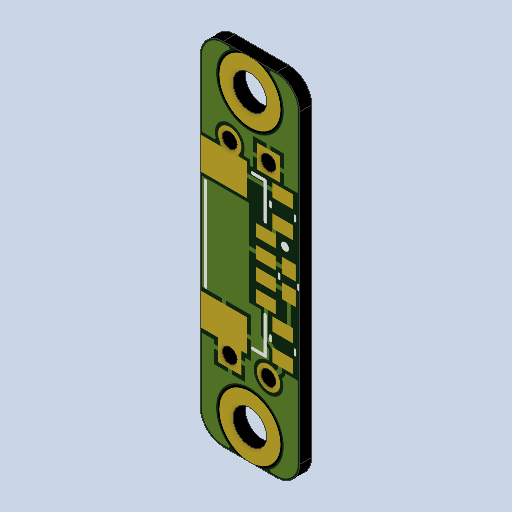
# Autodesk Inventor part: ND.ForageFeeder.BeamBreak_BOARD
Saved by Autodesk Inventor 2023.2 (Build 272271000, 271)
## iProperties
Created: 2021-12-10
Part Number: ND.ForageFeeder.BeamBreak_BOARD
Material: Generic
Document SubType Name: Modeling
Designer: Graeme
Density: 1 g/cm^3
Appearance: BoardColor
Author: Graeme
Autodesk Inventor part; units mm, degrees
ref_plane "YZ Plane" through (0, 0, 0) normal (1, 0, 0) x (0, 1, 0)
ref_plane "XZ Plane" through (0, 0, 0) normal (0, 1, 0) x (-1, 0, 0)
ref_plane "BoardFrontPlane" through (0, 0, 0) normal (0, 0, 1) x (1, 0, 0)
sketch "Sketch1" plane through (0, 0, 0) normal (0, 0, 1) x (1, 0, 0)
  line L0 (24, 22.5) -> (24, 42.5)
  arc A0 (25.5, 44) -> (24, 42.5) centre (25.5, 42.5) ccw
  line L1 (25.5, 44) -> (29, 44)
  arc A1 (30.5, 42.5) -> (29, 44) centre (29, 42.5) ccw
  line L2 (30.5, 42.5) -> (30.5, 22.5)
  arc A2 (29, 21) -> (30.5, 22.5) centre (29, 22.5) ccw
  line L3 (29, 21) -> (25.5, 21)
  arc A3 (24, 22.5) -> (25.5, 21) centre (25.5, 22.5) ccw
  constraints: 8 end point, 8 point on circle, 4 centre point
extrude "BoardOutline" add sketch "Sketch1" along normal blind 0.798
sketch "img_Top" plane through (0, 0, 0.798) normal (0, 0, 1) x (1, 0, 0)
  line L0 (24, 44) -> (30.4988, 44) construction
  line L1 (30.4988, 44) -> (30.4988, 21) construction
  line L2 (30.4988, 21) -> (24, 21) construction
  line L3 (24, 21) -> (24, 44) construction
  constraints: 2 other
decal "Decal_Top"
sketch "img_Bottom" plane through (0, 0, -0.798) normal (0, 0, -1) x (1, 0, 0)
  line L0 (24, -21) -> (30.4988, -21) construction
  line L1 (30.4988, -21) -> (30.4988, -44) construction
  line L2 (30.4988, -44) -> (24, -44) construction
  line L3 (24, -44) -> (24, -21) construction
  constraints: 2 other
decal "Decal_Bottom"
sketch "Sketch4" plane through (0, 0, 0.798) normal (0, 0, 1) x (1, 0, 0)
  point P0 (28.47, 26.4)
hole "Q1-2" at (28.47, 26.4, 0.798) direction (0, 0, -1) diameter 0.9652 end through all
sketch "Sketch5" plane through (0, 0, 0.798) normal (0, 0, 1) x (1, 0, 0)
  point P0 (25.93, 26.4)
hole "Q1-1" at (25.93, 26.4, 0.798) direction (0, 0, -1) diameter 0.9652 end through all
sketch "Sketch6" plane through (0, 0, 0.798) normal (0, 0, 1) x (1, 0, 0)
  point P0 (28.47, 38.6)
hole "LED1-1" at (28.47, 38.6, 0.798) direction (0, 0, -1) diameter 0.9652 end through all
sketch "Sketch7" plane through (0, 0, 0.798) normal (0, 0, 1) x (1, 0, 0)
  point P0 (25.93, 38.6)
hole "LED1-2" at (25.93, 38.6, 0.798) direction (0, 0, -1) diameter 0.9652 end through all
sketch "Sketch8" plane through (0, 0, 0.798) normal (0, 0, 1) x (1, 0, 0)
  point P0 (27.25, 42)
hole "Free-MP2" at (27.25, 42, 0.798) direction (0, 0, -1) diameter 2.2 end through all
sketch "Sketch9" plane through (0, 0, 0.798) normal (0, 0, 1) x (1, 0, 0)
  point P0 (27.25, 23)
hole "Free-MP1" at (27.25, 23, 0.798) direction (0, 0, -1) diameter 2.2 end through all
body "Solid1"
